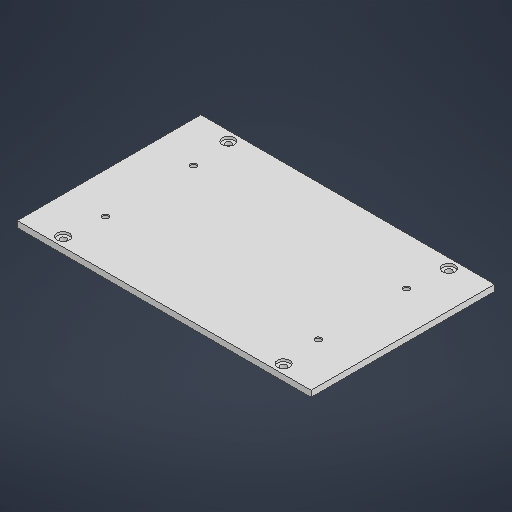
# Autodesk Inventor part: Hotplate Mount
Saved by Autodesk Inventor 2025.1 (Build 291241000, 241)
## iProperties
Created: 2025-02-19
Part Number: Hotplate Mount
Material: Generic
Document SubType Name: Modeling
Designer: jerem
Density: 1 g/cm^3
Appearance: Default
Author: jerem
Autodesk Inventor part; units mm, degrees
ref_plane "YZ Plane" through (0, 0, 0) normal (1, 0, 0) x (0, 1, 0)
ref_plane "XZ Plane" through (0, 0, 0) normal (0, 1, 0) x (-1, 0, 0)
ref_plane "XY Plane" through (0, 0, 0) normal (0, 0, 1) x (1, 0, 0)
sketch "Sketch1" plane through (0, 0, 0) normal (0, 1, 0) x (-1, 0, 0)
  line L0 (-120, -75) -> (120, -75)
  line L1 (120, -75) -> (120, 75)
  line L2 (120, 75) -> (-120, 75)
  line L3 (-120, 75) -> (-120, -75)
  line L4 (-120, -75) -> (120, 75) construction
  line L5 (120, -75) -> (-120, 75) construction
  point P0 (0, 0)
  dimension "d0" = 240
  dimension "d1" = 150
  constraints: 12 end point, 2 midpoint, 2 parallel, 1 horizontal, 1 perpendicular
  measures "d0" distance of L1.end L2.end
  measures "d1" distance of L0.end L1.end
extrude "Extrusion1" add sketch "Sketch1" along normal blind 5
sketch "Sketch2" plane through (0, 0, 0) normal (0, 1, 0) x (1, 0, 0)
  line L0 (-120, 75) -> (-120, -75) projected
  line L1 (-120, -75) -> (120, -75) projected
  line L2 (120, -75) -> (120, 75) projected
  line L3 (120, 75) -> (-120, 75) projected
  line L4 (-87, -36) -> (87, -36) construction
  line L5 (87, -36) -> (87, 36) construction
  line L6 (87, 36) -> (-87, 36) construction
  line L7 (-87, 36) -> (-87, -36) construction
  line L8 (-120, 0) -> (-87, 0) construction
  line L9 (0, 36) -> (0, 75) construction
  line L10 (0, -36) -> (0, -75) construction
  line L11 (87, 0) -> (120, 0) construction
  point P0 (0, 0)
  dimension "d4" = 72
  dimension "d5" = 174
  constraints: 16 end point, 8 midpoint, 4 coincident, 3 perpendicular, 2 parallel, 1 horizontal
  measures "d4" distance of L6.end L4.start
  measures "d5" distance of L4.start L4.end
hole "Hole1" at (-87, 0, 36) at (-87, 0, -36) at (87, 0, -36) at (87, 0, 36) direction (0, 1, 0) diameter 5 end through all counterbore diameter 10 counterbore depth 4
sketch "Sketch3" plane through (0, 5, 0) normal (0, 1, 0) x (1, 0, 0)
  line L0 (-90, -67.5) -> (90, -67.5) construction
  line L1 (90, -67.5) -> (90, 67.5) construction
  line L2 (90, 67.5) -> (-90, 67.5) construction
  line L3 (-90, 67.5) -> (-90, -67.5) construction
  line L4 (-90, -67.5) -> (90, 67.5) construction
  line L5 (90, -67.5) -> (-90, 67.5) construction
  point P0 (0, 0)
  dimension "d13" = 180
  dimension "d14" = 135
  constraints: 12 end point, 4 coincident, 2 midpoint, 2 parallel, 1 horizontal, 1 perpendicular
  measures "d13" distance of L2.end L1.end
  measures "d14" distance of L1.end L0.end
hole "Hole2" at (90, 5, -67.5) at (90, 5, 67.5) at (-90, 5, 67.5) at (-90, 5, -67.5) direction (0, -1, 0) diameter 5 end through all counterbore diameter 10 counterbore depth 2
body "Solid1"
